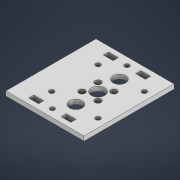
# Autodesk Inventor part: pumpeplade
Saved by Autodesk Inventor 2022 (Build 260153000, 153)
## iProperties
Created: 2022-03-02
Part Number: pumpeplade
Material: Generic
Document SubType Name: Modeling
Designer: Jakob Saugbjerg
Density: 1 g/cm^3
Appearance: Default
Author: Jakob Saugbjerg
Autodesk Inventor part; units mm, degrees
ref_plane "YZ Plane" through (0, 0, 0) normal (1, 0, 0) x (0, 1, 0)
ref_plane "XZ Plane" through (0, 0, 0) normal (0, 1, 0) x (-1, 0, 0)
ref_plane "XY Plane" through (0, 0, 0) normal (0, 0, 1) x (1, 0, 0)
sketch "Sketch1" plane through (0, 0, 0) normal (0, 1, 0) x (-1, 0, 0)
  line L0 (0, 0) -> (52, 0)
  line L1 (52, 0) -> (52, 60)
  line L2 (52, 60) -> (0, 60)
  line L3 (0, 60) -> (0, 0)
  dimension "d0" = 52
  dimension "d1" = 60
  constraints: 8 end point, 2 parallel, 1 horizontal, 1 perpendicular
  measures "d0" distance of L2.end L1.end
  measures "d1" distance of L1.end L0.end
extrude "Extrusion1" add sketch "Sketch1" along normal blind 3
sketch "Sketch2" plane through (0, 3, 0) normal (0, 1, 0) x (1, 0, 0)
  line L0 (-52, 0) -> (-52, -60) projected
  line L1 (-52, 0) -> (-40.2, 0)
  line L2 (-40.2, 0) -> (-40.2, -3.4)
  line L3 (-40.2, -3.4) -> (-52, -3.4)
  line L4 (-52, -3.4) -> (-52, 0)
  line L5 (-40.2, -3.4) -> (-33.7, -3.4)
  line L6 (-33.7, -3.4) -> (-33.7, -6.9)
  line L7 (-33.7, -6.9) -> (-40.2, -6.9)
  line L8 (-40.2, -6.9) -> (-40.2, -3.4)
  line L9 (-33.7, -3.4) -> (-18.7, -3.4)
  line L10 (-18.7, -3.4) -> (-12.2, -3.4)
  line L11 (-12.2, -3.4) -> (-12.2, -6.9)
  line L12 (-12.2, -6.9) -> (-18.7, -6.9)
  line L13 (-18.7, -6.9) -> (-18.7, -3.4)
  line L14 (-52, -30) -> (0, -30)
  line L15 (0, -60) -> (0, 0) projected
  line L16 (-40.2, -56.6) -> (-33.7, -56.6)
  line L17 (-33.7, -56.6) -> (-33.7, -53.1)
  line L18 (-33.7, -53.1) -> (-40.2, -53.1)
  line L19 (-40.2, -53.1) -> (-40.2, -56.6)
  line L20 (-18.7, -56.6) -> (-12.2, -56.6)
  line L21 (-12.2, -56.6) -> (-12.2, -53.1)
  line L22 (-12.2, -53.1) -> (-18.7, -53.1)
  line L23 (-18.7, -53.1) -> (-18.7, -56.6)
  dimension "d4" = 11.8
  dimension "d5" = 3.4
  dimension "d6" = 6.5
  dimension "d7" = 3.5
  dimension "d8" = 15
  dimension "d9" = 6.5
  dimension "d10" = 3.5
  constraints: 44 end point, 8 symmetric about line, 6 parallel, 4 horizontal, 3 perpendicular, 2 midpoint
  measures "d4" distance of L2.end L3.end
  measures "d5" distance of L1.end L2.end
  measures "d6" distance of L6.end L7.end
  measures "d7" distance of L5.end L6.end
  measures "d8" distance of L5.end L9.end
  measures "d9" distance of L11.end L12.end
  measures "d10" distance of L10.end L11.end
extrude "Extrusion2" cut sketch "Sketch2" against normal blind 3 contours L10 L11 L12 L13 | L5 L6 L7 L8 | L19 L18 L17 L16 | L23 L22 L21 L20
sketch "Sketch3" plane through (0, 3, 0) normal (0, 1, 0) x (1, 0, 0)
  line L0 (-52, -60) -> (0, -60) projected
  line L1 (-52, -60) -> (-20.9, -60)
  line L2 (-20.9, -60) -> (-20.9, -44.5)
  line L3 (-20.9, -44.5) -> (-52, -44.5)
  line L4 (-52, -44.5) -> (-52, -60)
  circle A0 centre (-20.9, -44.5) radius 4.25
  line L5 (-52, 0) -> (-52, -60) projected
  line L6 (-52, -30) -> (0, -30)
  line L7 (0, -60) -> (0, 0) projected
  circle A1 centre (-20.9, -15.5) radius 4.25
  dimension "d13" = 31.1
  dimension "d14" = 15.5
  dimension "d15" = 8.5
  constraints: 10 end point, 2 centre point, 2 midpoint, 2 parallel, 1 coincident, 1 horizontal, 1 perpendicular, 1 symmetric about line, 1 other
  measures "d13" distance of L3.end L2.end
  measures "d14" distance of L2.end L1.end
  measures "d15" diameter of A0
extrude "Extrusion3" cut sketch "Sketch3" against normal blind 3 contours A0 L3 L2 | L2 L3 A0 | A1
sketch "Sketch4" plane through (0, 3, 0) normal (0, 1, 0) x (1, 0, 0)
  circle A0 centre (-20.9, -44.5) radius 4.25 projected
  line L0 (-20.9, -40.25) -> (-20.9, -29.75)
  circle A1 centre (-20.9, -29.75) radius 4.5
  point P0 (0, 0)
  dimension "d18" = 10.5
  dimension "d19" = 9
  constraints: 2 end point, 1 centre point, 1 coincident, 1 vertical, 1 vertical alignment, 1 other
  measures "d18" distance of L0.start L0.end
  measures "d19" diameter of A1
extrude "Extrusion4" cut sketch "Sketch4" against normal blind 3 contours A1
sketch "Sketch5" plane through (0, 3, 0) normal (0, 1, 0) x (1, 0, 0)
  circle A0 centre (-20.9, -29.75) radius 4.5 projected
  line L0 (-20.9, -29.75) -> (-26.2033, -35.0533)
  line L1 (-20.9, -29.75) -> (-13.4, -29.75) construction
  circle A1 centre (-26.2033, -35.0533) radius 2.05
  point P0 (0, 0)
  dimension "d22" = 7.5
  dimension "d23" = 135
  dimension "d24" = 4.1
  constraints: 4 end point, 1 centre point, 1 coincident, 1 equal length, 1 horizontal
  measures "d22" distance of L0.start L0.end
  measures "d23" angle of L0 L1
  measures "d24" diameter of A1
extrude "Extrusion5" cut sketch "Sketch5" against normal blind 3 contours A1
pattern_circular "Circular Pattern1" count 4 over 360 about axis through (-20.9, 3, 29.75) along (0, -1, 0) of "Extrusion5"
sketch "Sketch6" plane through (0, 3, 0) normal (0, 1, 0) x (1, 0, 0)
  circle A0 centre (-20.9, -29.75) radius 4.5 projected
  line L0 (-20.9, -29.75) -> (-5.4497, -45.2003)
  line L1 (-20.9, -29.75) -> (0.95, -29.75) construction
  circle A1 centre (-5.4497, -45.2003) radius 1.6
  line L2 (-20.9, -29.75) -> (-5.4497, -14.2997)
  line L3 (-20.9, -29.75) -> (-36.3503, -45.2003)
  line L4 (-20.9, -29.75) -> (-36.3503, -14.2997)
  circle A2 centre (-36.3503, -45.2003) radius 1.6
  circle A3 centre (-36.3503, -14.2997) radius 1.6
  circle A4 centre (-5.4497, -14.2997) radius 1.6
  point P0 (0, 0)
  dimension "d30" = 21.85
  dimension "d31" = 45
  dimension "d32" = 3.2
  dimension "d35" = 21.85
  dimension "d36" = 21.85
  dimension "d37" = 21.85
  dimension "d38" = 3.2
  dimension "d39" = 3.2
  dimension "d40" = 3.2
  constraints: 10 end point, 4 centre point, 4 coincident, 1 equal length, 1 horizontal
  measures "d30" distance of L0.start L0.end
  measures "d31" angle of L0 L1
  measures "d32" diameter of A1
  measures "d35" distance of L0.start L2.end
  measures "d36" distance of L0.start L3.end
  measures "d37" distance of L0.start L4.end
  measures "d38" diameter of A2
  measures "d39" diameter of A3
  measures "d40" diameter of A4
extrude "Extrusion6" cut sketch "Sketch6" against normal blind 3.2 contours A1 | A2 | A3 | A4
sketch "Sketch7" plane through (0, 3, 0) normal (0, 1, 0) x (1, 0, 0)
  line L0 (-33.7, -6.9) -> (-33.7, -3.4) projected
  line L1 (-33.7, -5.15) -> (-26.2, -5.15)
  line L2 (-52, 0) -> (-52, -60) projected
  line L3 (-52, -30) -> (-2, -30)
  circle A0 centre (-26.2, -5.15) radius 1.55
  circle A1 centre (-26.2, -54.85) radius 1.55
  point P0 (0, 0)
  dimension "d41" = 7.5
  dimension "d42" = 50
  dimension "d43" = 3.1
  constraints: 4 end point, 2 centre point, 2 horizontal, 2 midpoint, 1 coincident, 1 symmetric about line, 1 other
  measures "d41" distance of L1.start L1.end
  measures "d42" distance of L3.start L3.end
  measures "d43" diameter of A0
extrude "Extrusion7" cut sketch "Sketch7" against normal blind 3.1
equation "\"d33\" = d39"
equation "\"d44\" = d43"
body "Solid1"
